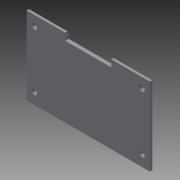
# Autodesk Inventor part: Enclosure-Backplate01
Saved by Autodesk Inventor 2015 (Build 190159000, 159)
## iProperties
Created: 2014-04-13
Part Number: Enclosure-Backplate01
Material: Generic
Document SubType Name: Modeling
Designer: spichelh
Density: 1 g/cm^3
Appearance: Default
Author: spichelh
Autodesk Inventor part; units mm, degrees
ref_plane "YZ Plane" through (0, 0, 0) normal (1, 0, 0) x (0, 1, 0)
ref_plane "XZ Plane" through (0, 0, 0) normal (0, 1, 0) x (-1, 0, 0)
ref_plane "XY Plane" through (0, 0, 0) normal (0, 0, 1) x (1, 0, 0)
sketch "Sketch1" plane through (0, 0, 0) normal (0, 0, 1) x (1, 0, 0)
  line L0 (107.6, 68) -> (107.6, 0)
  line L1 (107.6, 0) -> (0, 0)
  line L2 (0, 0) -> (0, 68)
  line L3 (0, 68) -> (33.75, 68)
  line L4 (33.75, 68) -> (33.75, 61.9)
  line L5 (33.75, 61.9) -> (73.85, 61.9)
  line L6 (73.85, 61.9) -> (73.85, 68)
  line L7 (73.85, 68) -> (107.6, 68)
  line L8 (53.8, 0) -> (53.8, -26.1159) construction
  line L9 (53.8, 61.9) -> (53.8, 35.6829) construction
  dimension "d37" = 40.1
  dimension "d38" = 107.6
  dimension "d39" = 68
  dimension "d64" = 6.1
  constraints: 28 end point, 4 collinear, 3 perpendicular, 2 horizontal, 2 midpoint, 2 parallel, 1 coincident, 1 vertical, 1 other
  measures "d37" distance of L4.end L5.end
  measures "d38" distance of L0.end L1.end
  measures "d39" distance of L1.end L2.end
  measures "d64" distance between parallel lines of L7 L5
extrude "Extrusion1" add sketch "Sketch1" along normal blind 3
sketch "Sketch4" plane through (0, 0, 0) normal (0, 0, -1) x (-1, 0, 0)
  line L0 (-33.75, 68) -> (0, 68) projected
  line L1 (-33.75, 61.9) -> (-33.75, 68) projected
  line L2 (-73.85, 61.9) -> (-33.75, 61.9) projected
  line L3 (-73.85, 68) -> (-73.85, 61.9) projected
  line L4 (-107.6, 68) -> (-73.85, 68) projected
  line L5 (-107.6, 0) -> (-107.6, 68) projected
  line L6 (0, 0) -> (-107.6, 0) projected
  line L7 (0, 68) -> (0, 0) projected
  line L8 (-71.25, 65.4) -> (-71.25, 63.4)
  line L9 (-71.25, 63.4) -> (-36.35, 63.4)
  line L10 (-36.35, 63.4) -> (-36.35, 65.4)
  line L11 (-36.35, 65.4) -> (-2.6, 65.4)
  line L12 (-71.25, 65.4) -> (-105, 65.4)
  line L13 (-105, 65.4) -> (-105, 2.6)
  line L14 (-2.6, 2.6) -> (-2.6, 65.4)
  line L15 (-105, 2.6) -> (-85.29, 2.6)
  line L16 (-85.29, 2.6) -> (-85.29, 5.1)
  line L17 (-85.29, 5.1) -> (-22.31, 5.1)
  line L18 (-22.31, 5.1) -> (-22.31, 2.6)
  line L19 (-22.31, 2.6) -> (-2.6, 2.6)
  line L20 (-53.8, 0) -> (-53.8, 2.6) construction
  line L21 (-53.8, 5.1) -> (-53.8, 2.6) construction
  dimension "d42" = 2.6
  dimension "d43" = 2.6
  dimension "d44" = 2.6
  dimension "d45" = 2.6
  dimension "d46" = 2.6
  dimension "d48" = 2.6
  dimension "d49" = 5.1
  dimension "d50" = 2.6
  dimension "d51" = 2.6
  dimension "d52" = 62.98
  dimension "d65" = 2
  constraints: 28 end point, 6 perpendicular, 4 parallel, 3 collinear, 2 midpoint, 1 horizontal, 1 vertical
  measures "d42" distance between parallel lines of L3 L8
  measures "d43" distance between parallel lines of L1 L10
  measures "d44" distance between parallel lines of L0 L11
  measures "d45" distance between parallel lines of L12 L4
  measures "d46" distance between parallel lines of L5 L13
  measures "d48" distance between parallel lines of L14 L7
  measures "d49" distance between parallel lines of L6 L17
  measures "d50" distance between parallel lines of L6 L15
  measures "d51" distance between parallel lines of L19 L6
  measures "d52" distance between parallel lines of L16 L18
  measures "d65" distance between parallel lines of L12 L9
extrude "Extrusion4" cut sketch "Sketch4" against normal blind 1 contours L0 L7 L6 L5 L4 L3 L12 L13 L15 L16 L17 L18 L19 L14 L11 L1
sketch "Sketch5" plane through (0, 0, 3) normal (0, 0, 1) x (1, 0, 0)
  circle A0 centre (6.8128, 9.8088) radius 1.5 projected
  circle A1 centre (6.81, 59.3388) radius 1.5 projected
  circle A2 centre (100.7928, 9.8142) radius 1.5 projected
  circle A3 centre (100.79, 59.3442) radius 1.5 projected
  line L0 (104.603, 6.0044) -> (3.003, 5.9986) projected
  line L1 (104.5998, 63.1544) -> (104.603, 6.0044) projected
  line L2 (2.9998, 63.1486) -> (104.5998, 63.1544) projected
  line L3 (3.003, 5.9986) -> (2.9998, 63.1486) projected
  circle A4 centre (6.81, 59.3388) radius 1.4
  circle A5 centre (6.8128, 9.8088) radius 1.4
  circle A6 centre (100.7928, 9.8142) radius 1.4
  circle A7 centre (100.79, 59.3442) radius 1.4
  point P0 (0, 0)
  dimension "d55" = 2.8
  dimension "d56" = 2.8
  dimension "d57" = 2.8
  dimension "d58" = 2.8
  constraints: 4 centre point, 4 coincident
  measures "d55" diameter of A4
  measures "d56" diameter of A5
  measures "d57" diameter of A6
  measures "d58" diameter of A7
extrude "Extrusion5" cut sketch "Sketch5" against normal blind 4 contours A4 | A5 | A6 | A7
chamfer "Chamfer3" distance 1 angle 45 4 edges at (5.41, 59.3388, 3) (5.4128, 9.8088, 3) (99.39, 59.3442, 3) (99.3928, 9.8142, 3)
body "Solid1"
